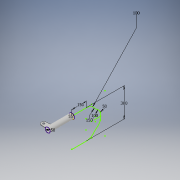
# Autodesk Inventor part: 前桿1
Saved by Autodesk Inventor 2019 (Build 230136000, 136)
## iProperties
Created: 2021-03-26
Part Number: 前桿1
Material: 一般
Document SubType Name: Modeling
Designer: cadlab
Density: 1 g/cm^3
Appearance: 預設
Author: cadlab
Autodesk Inventor part; units mm, degrees
ref_plane "YZ Plane" through (0, 0, 0) normal (1, 0, 0) x (0, 1, 0)
ref_plane "XY Plane" through (0, 0, 0) normal (0, 0, 1) x (1, 0, 0)
sketch "草圖3" plane through (0, 0, 0) normal (0, 0, 1) x (1, 0, 0)
  circle A0 centre (0, 0) radius 25
  dimension "d5" = 50
  constraints: 1 centre point, 1 coincident
  measures "d5" diameter of A0
extrude "擠出1" add sketch "草圖3" against normal blind 250
sketch "草圖4" plane through (0, 0, 0) normal (0, 1, 0) x (-1, 0, 0)
  line L0 (-25, 0) -> (25, 0) projected
  circle A0 centre (75, -35) radius 10
  arc A1 (75, -60) -> (75, -10) centre (75, -35) ccw
  line L1 (75, -60) -> (29.5025, -64.5498)
  line L2 (25, 0) -> (25, -0.4751)
  line L3 (75, -10) -> (29.5025, -5.4502)
  arc A2 (25, -0.4751) -> (29.5025, -5.4502) centre (30, -0.4751) ccw
  arc A3 (29.5025, -64.5498) -> (25, -69.5249) centre (30, -69.5249) ccw
  line L4 (25, -0.4751) -> (25, -69.5249)
  point P0 (0, 0)
  point P1 (25, -5)
  dimension "d21" = 20
  dimension "d28" = 25
  dimension "d31" = 5
  dimension "d32" = 50
  dimension "d33" = 50
  dimension "d34" = 25
  constraints: 8 end point, 6 point on circle, 4 centre point, 3 tangent, 2 point on line, 1 coincident
  measures "d21" diameter of A0
  measures "d28" distance of L3.start A0.centre
  measures "d31" radius of A2
  measures "d32" horizontal distance of L2.end L3.start
  measures "d33" horizontal distance of L0.end A0.centre
  measures "d34" radius of A1
extrude "擠出2" add sketch "草圖4" along normal mid plane 5
sketch "草圖7" plane through (0, 0, 0) normal (1, 0, 0) x (0, 1, 0)
  line L0 (-25, -250) -> (25, -250) projected
  line L1 (0, -400) -> (0, -250)
  arc A0 (-38.2176, -478.6316) -> (-68.2176, -510.2588) centre (54.456, -596.5791) ccw
  line L2 (-150, -479.8436) -> (-150, -554.8436)
  arc A1 (-103.2189, -541.0949) -> (-68.2176, -510.2588) centre (-150, -452.712) ccw
  line L3 (-150, -546.9034) -> (-126.6094, -546.9034)
  arc A2 (-126.6094, -546.9034) -> (-103.2189, -541.0949) centre (-126.6094, -496.9034) ccw
  arc A3 (-38.2176, -478.6316) -> (0, -400) centre (-100, -400) ccw
  line L4 (-300, -400) -> (-300, -250)
  arc A4 (-231.7824, -510.2588) -> (-261.7824, -478.6316) centre (-354.456, -596.5791) ccw
  arc A5 (-231.7824, -510.2588) -> (-196.7811, -541.0949) centre (-150, -452.712) ccw
  line L5 (-150, -546.9034) -> (-173.3906, -546.9034)
  arc A6 (-196.7811, -541.0949) -> (-173.3906, -546.9034) centre (-173.3906, -496.9034) ccw
  arc A7 (-300, -400) -> (-261.7824, -478.6316) centre (-200, -400) ccw
  line L6 (0, -400) -> (0, -250)
  point P0 (0, 0)
  point P1 (0, -250)
  point P2 (0, -456.8131)
  point P3 (-116.4146, -546.9034)
  point P4 (-300, -250)
  point P5 (-300, -456.8131)
  point P6 (-183.5854, -546.9034)
  dimension "d114" = 100
  dimension "d115" = 50
  dimension "d116" = 100
  dimension "d118" = 150
  dimension "d127" = 300
  dimension "d139" = 150
  constraints: 20 point on circle, 12 end point, 10 symmetric about line, 8 centre point, 5 tangent, 4 point on line, 2 vertical, 1 midpoint, 4 other
  measures "d114" radius of A1
  measures "d115" radius of A2
  measures "d116" radius of A3
  measures "d118" radius of A0
  measures "d127" distance of L4.start L1.start
  measures "d139" distance of L1.start point (0, -250)
ref_plane "工作平面14" through (0, 0, -250) normal (0, 0, -1) x (-1, 0, 0)
sketch "草圖26" plane through (0, 0, -250) normal (0, 0, -1) x (-1, 0, 0)
  circle A0 centre (0, 0) radius 25 projected
  circle A1 centre (0, 0) radius 27.5
  dimension "d117" = 55
  constraints: 1 centre point, 1 coincident
  measures "d117" diameter of A1
sketch "草圖27" plane through (0, -150, -546.9034) normal (0, 0, -1) x (-1, 0, 0)
  circle A0 centre (0, 0) radius 17.5
  point P0 (0, 150)
  dimension "d119" = 35
  constraints: 1 centre point
  measures "d119" diameter of A0
sketch "草圖29" plane through (0, 0, -250) normal (0, 0, -1) x (-1, 0, 0)
  circle A0 centre (0, -300) radius 25
  point P0 (0, 0)
  dimension "d124" = 50
  constraints: 1 centre point, 1 coincident
  measures "d124" diameter of A0
sketch "草圖30" plane through (0, -300, 0) normal (0, 1, 0) x (-1, 0, 0)
  arc A0 (25, -0.4751) -> (29.5025, -5.4502) centre (30, -0.4751) ccw projected
  line L0 (25, -69.5249) -> (25, -69)
  arc A1 (75, -60) -> (75, -10) centre (75, -35) ccw projected
  line L1 (29.5025, -64.5498) -> (75, -60) projected
  line L2 (25, -0.4751) -> (25, -69.5249) projected
  circle A2 centre (75, -35) radius 10
  arc A3 (75, -60) -> (75, -10) centre (75, -35) ccw
  line L3 (75, -60) -> (29.5025, -64.5498)
  line L4 (25, -10) -> (25, -5)
  line L5 (75, -10) -> (29.5025, -5.4502) projected
  line L6 (29.5025, -5.4502) -> (75, -10)
  arc A4 (29.5025, -64.5498) -> (25, -69.5249) centre (30, -69.5249) ccw
  line L7 (25, -0.4751) -> (25, -0.4751)
  arc A5 (25, -0.4751) -> (29.5025, -5.4502) centre (30, -0.4751) ccw
  point P0 (0, 0)
  point P1 (25, -65)
  dimension "d129" = 50
  dimension "d130" = 5
  dimension "d131" = 5
  dimension "d132" = 5
  constraints: 11 end point, 6 point on circle, 6 point on line, 6 tangent, 4 centre point, 2 coincident, 2 vertical, 1 collinear, 1 concentric
  measures "d129" distance of L5.start L4.start
  measures "d130" distance of L4.start L4.end
  measures "d131" radius of A4
  measures "d132" radius of A5
